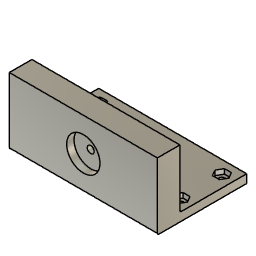
Soporte cámara individual (Parte trasera) (Autodesk Fusion 360 design; units mm, degrees)
part number: Configuracion 1
Autodesk Fusion 360 part; units mm, degrees
sketch "Boceto1" plane through (0, 0, 0) normal (0, 0, 1) x (1, 0, 0)
  line L0 (24.6, -11.1) -> (-24.6, -11.1)
  line L1 (-24.6, -11.1) -> (-24.6, 11.1)
  line L2 (-24.6, 11.1) -> (24.6, 11.1)
  line L3 (24.6, 11.1) -> (24.6, -11.1)
  line L4 (24.6, -11.1) -> (-24.6, 11.1) construction
  line L5 (-24.6, -11.1) -> (24.6, 11.1) construction
  circle A0 centre (-20.59, 6.89) radius 1
  line L6 (-24.6, 0) -> (24.6, 0) construction
  circle A1 centre (-20.59, -6.89) radius 1
  line L7 (-20.59, 6.89) -> (-20.59, -6.89) construction
  line L8 (0, 11.1) -> (0, -11.1) construction
  circle A2 centre (20.59, 6.89) radius 1
  circle A3 centre (20.59, -6.89) radius 1
  line L9 (24.6, -18.6) -> (-24.6, -18.6)
  line L10 (-24.6, -18.6) -> (-24.6, -11.1)
  line L11 (-24.6, -11.1) -> (24.6, -11.1)
  line L12 (24.6, -11.1) -> (24.6, -18.6)
  line L13 (24.6, -18.6) -> (-24.6, -11.1) construction
  line L14 (-24.6, -18.6) -> (24.6, -11.1) construction
  point P0 (-20.59, -5.89)
  point P1 (-20.59, 5.89)
  point P2 (0, -14.85)
  dimension "d1" = 22.2
  dimension "d2" = 49.2
  dimension "d3" = 2
  dimension "d4" = 4.01
  dimension "d5" = 4.21
  dimension "d10" = 49.2
  dimension "d11" = 7.5
  constraint horizontal L0
  constraint perpendicular L0 L1
  constraint parallel L0 L2
  constraint parallel L1 L3
  constraint coincident L4 origin
  constraint coincident L5 origin
  constraint midpoint L1 L6.start
  constraint midpoint L3 L6.end
  constraint symmetric A0 L6 A1
  constraint coincident A0.centre L7.start
  constraint coincident A1.centre L7.end
  constraint coincident A1 P0
  constraint coincident L7 P0
  constraint coincident A0 P1
  constraint coincident L7 P1
  constraint midpoint L2 L8.start
  constraint midpoint L0 L8.end
  constraint symmetric A0 L8 A2
  constraint symmetric A1 L8 A3
  constraint horizontal L9
  constraint perpendicular L9 L10
  constraint parallel L9 L11
  constraint parallel L10 L12
  constraint coincident L13 P2
  constraint coincident L14 P2
  constraint collinear L0 L11
  constraint collinear L3 L12
  measures "d1" distance of L0.end L1.end
  measures "d2" distance of L1.end L2.end
  measures "d3" diameter of A0
  measures "d4" distance of L1 A0.centre
  measures "d5" distance of L2 A0.centre
  measures "d10" distance of L0.end L0.start
  measures "d11" distance of L9.end L0.end
extrude "Extruir1" add sketch "Boceto1" along normal blind 2.8 contours L0 L1 L2 L3 L11
extrude "Extruir2" add sketch "Boceto1" along normal blind 22.2 contours L0 L9 L10 L11 L12
fillet "Empalme1" radius 0.5 1 edges at (0, -11.1, 2.8)
sketch "Boceto2" plane through (0, -18.6, 0) normal (0, -1, 0) x (1, 0, 0)
  line L0 (-24.6, 0) -> (24.6, 0)
  line L1 (24.6, 0) -> (24.6, 22.2)
  line L2 (24.6, 22.2) -> (-24.6, 22.2)
  line L3 (-24.6, 22.2) -> (-24.6, 0)
  circle A0 centre (0, 11.1) radius 5.55
  line L4 (-24.6, 11.1) -> (24.6, 11.1) construction
  circle A1 centre (0, 11.1) radius 1.175
  dimension "d20" = 11.1
  dimension "d21" = 2.35
  constraint coincident L3 L4.start
  constraint midpoint L1 L4.end
  constraint perpendicular L1 L4
  constraint midpoint A0.centre L4
  constraint concentric A0 A1
  measures "d20" diameter of A0
  measures "d21" diameter of A1
extrude "Extruir3" cut sketch "Boceto2" against normal blind 2.45 contours A0
extrude "Extruir4" cut sketch "Boceto2" against normal blind 4.9 contours A1
sketch "Boceto3" plane through (0, 0, 2.8) normal (0, 0, 1) x (-1, 0, 0)
  line L0 (24.6, 10.6) -> (-24.6, 10.6)
  line L1 (-24.6, 10.6) -> (-24.6, -11.1)
  line L2 (-24.6, -11.1) -> (24.6, -11.1)
  line L3 (24.6, -11.1) -> (24.6, 10.6)
  circle A0 centre (-20.59, -6.89) radius 1
  circle A1 centre (20.59, -6.89) radius 1
  circle A2 centre (20.59, 6.89) radius 1
  circle A3 centre (-20.59, 6.89) radius 1
  line L4 (-19.4353, -8.89) -> (-18.2806, -6.89)
  line L5 (-18.2806, -6.89) -> (-19.4353, -4.89)
  line L6 (-19.4353, -4.89) -> (-21.7447, -4.89)
  line L7 (-21.7447, -4.89) -> (-22.8994, -6.89)
  line L8 (-22.8994, -6.89) -> (-21.7447, -8.89)
  line L9 (-21.7447, -8.89) -> (-19.4353, -8.89)
  line L10 (0, 10.6) -> (0, -11.1) construction
  line L11 (-18.2806, 6.89) -> (-19.4353, 8.89)
  line L12 (-19.4353, 8.89) -> (-21.7447, 8.89)
  line L13 (-21.7447, 8.89) -> (-22.8994, 6.89)
  line L14 (-22.8994, 6.89) -> (-21.7447, 4.89)
  line L15 (-21.7447, 4.89) -> (-19.4353, 4.89)
  line L16 (-19.4353, 4.89) -> (-18.2806, 6.89)
  line L17 (21.7447, -8.89) -> (19.4353, -8.89)
  line L18 (19.4353, -8.89) -> (18.2806, -6.89)
  line L19 (18.2806, -6.89) -> (19.4353, -4.89)
  line L20 (22.8994, -6.89) -> (21.7447, -8.89)
  line L21 (21.7447, -4.89) -> (22.8994, -6.89)
  line L22 (19.4353, -4.89) -> (21.7447, -4.89)
  line L23 (21.7447, 4.89) -> (19.4353, 4.89)
  line L24 (19.4353, 4.89) -> (18.2806, 6.89)
  line L25 (18.2806, 6.89) -> (19.4353, 8.89)
  line L26 (19.4353, 8.89) -> (21.7447, 8.89)
  line L27 (21.7447, 8.89) -> (22.8994, 6.89)
  line L28 (22.8994, 6.89) -> (21.7447, 4.89)
  point P0 (-20.59, -6.89)
  point P1 (-20.59, 6.89)
  dimension "d26" = 2
  dimension "d27" = 2
  constraint horizontal L6
  constraint coincident P0 A0.centre
  constraint midpoint L0 L10.start
  constraint midpoint L2 L10.end
  constraint coincident P1 A3.centre
  constraint horizontal L12
  constraint symmetric L4.start L10 L17.end
  constraint symmetric L4.end L10 L18.end
  constraint symmetric L5.end L10 L19.end
  constraint symmetric L6.end L10 L21.start
  constraint symmetric L7.end L10 L20.start
  constraint symmetric L8.end L10 L17.start
  constraint symmetric L10 L11.start L24.end
  constraint symmetric L10 L11.end L25.end
  constraint symmetric L10 L12.end L26.end
  constraint symmetric L10 L13.end L27.end
  constraint symmetric L10 L14.end L23.start
  constraint symmetric L10 L15.end L23.end
  measures "d26" distance of P0 L9
  measures "d27" distance of P1 L16
extrude "Extruir5" cut sketch "Boceto3" against normal blind 1.6 contours L4 L5 L6 L7 L8 L9 | L11 L12 L13 L14 L15 L16 | L17 L18 L19 L20 L21 L22 | L23 L24 L25 L26 L27 L28
fillet "Empalme3" radius 0.5 1 edges at (0, -18.6, 0)
equation "d1 = 18 mm + tolerancia * 2 + grosor2 * 2"
equation "d2 = 45 mm + tolerancia * 2 + grosor2 * 2"
equation "d3 = 1.9 mm + tolerancia"
equation "d4 = 1.91 mm + grosor2 + tolerancia"
equation "d5 = 2.11 mm + grosor2 + tolerancia"
equation "grosor1 = 2.8 mm"
equation "grosor2 = 2 mm"
equation "grosor3 = 7.5 mm"
equation "tolerancia = 0.1 mm"
equation "d10 = d2"
equation "d11 = grosor3"
equation "d12 = grosor1"
equation "d14 = d1"
equation "d20 = 11 mm + tolerancia"
equation "d21 = 2.25 mm + tolerancia"
